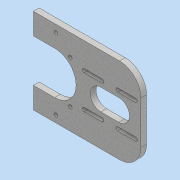
# Autodesk Inventor part: Uchwyt silnika krokowego osi Zi
Saved by Autodesk Inventor 2018 (Build 220112000, 112)
## iProperties
Created: 2019-02-03
Part Number: Uchwyt silnika krokowego osi Zi
Material: Ogólny
Document SubType Name: Modeling
Designer: Dawid
Density: 1 g/cm^3
Appearance: Aluminium odlewane
Author: Dawid
Autodesk Inventor part; units mm, degrees
ref_plane "YZ Plane" through (0, 0, 0) normal (1, 0, 0) x (0, 1, 0)
ref_plane "XZ Plane" through (0, 0, 0) normal (0, 1, 0) x (-1, 0, 0)
ref_plane "XY Plane" through (0, 0, 0) normal (0, 0, 1) x (1, 0, 0)
sketch "Szkic1" plane through (0, 0, 0) normal (0, 1, 0) x (-1, 0, 0)
  line L0 (-28, -60) -> (29, -60)
  line L1 (-28, 60) -> (29, 60)
  line L2 (-28, 60) -> (-36, 60)
  line L3 (-36, -60) -> (-28, -60)
  circle A0 centre (-81, 0) radius 12.5
  circle A1 centre (0, 0) radius 24
  line L4 (-111, -60) -> (-36, -60)
  line L5 (-111, 60) -> (-36, 60)
  line L6 (29, 60) -> (29, -60)
  line L7 (-31, -30) -> (29, -30)
  line L8 (-31, 30) -> (29, 30)
  circle A2 centre (-81, 0) radius 15
  line L9 (-116, -60) -> (-111, -60)
  line L10 (-116, 60) -> (-111, 60)
  line L11 (-116, -60) -> (-119.57, -60)
  line L12 (-119.57, 60) -> (-116, 60)
  line L13 (-119.57, -60) -> (-122.07, -60)
  line L14 (-122.07, -60) -> (-122.07, 60)
  line L15 (-122.07, 60) -> (-119.57, 60)
  line L16 (-31, -30) -> (-31, 30)
  dimension "d0" = 30
  constraints: 34 end point, 4 perpendicular, 3 centre point, 3 horizontal, 2 point on line, 1 coincident, 1 collinear, 1 vertical
  measures "d0" diameter of A2
extrude "Wyciągnięcie proste1" add sketch "Szkic1" along normal blind 8 contours L3 L4 L9 L11 L13 L14 L15 L12 L10 L5 L2 L1 L6 L8 L16 L7 L0
sketch "Szkic3" plane through (0, 8, 0) normal (0, 1, 0) x (1, 0, 0)
  line L0 (81, 15) -> (111, 15)
  line L1 (81, -15) -> (111, -15)
  arc A0 (11, -30) -> (11, 30) centre (11, 0) ccw projected
  circle A1 centre (81, 0) radius 15 projected
  arc A2 (66, 15) -> (66, -15) centre (66, 0) ccw
  line L2 (81, 15) -> (66, 15)
  line L3 (81, -15) -> (66, -15)
  arc A3 (91, -15) -> (91, 15) centre (91, 0) ccw
  line L4 (116, -60) -> (116, 60) projected
  line L5 (111, 15) -> (116, 15)
  line L6 (111, -15) -> (116, -15)
  point P0 (0, 0)
  point P1 (116, -30)
  point P2 (116, 30)
  constraints: 12 end point, 5 point on circle, 5 point on line, 2 centre point, 2 perpendicular, 1 parallel, 1 tangent
extrude "Wyciągnięcie proste4" cut sketch "Szkic3" against normal up to next contours L0 A3 L1 A1 | A1 | A1 L3 A2 L2
sketch "Szkic4" plane through (0, 8, 0) normal (0, 1, 0) x (1, 0, 0)
  line L0 (86, -60) -> (-29, -60)
  line L1 (-29, -60) -> (-29, -30)
  line L2 (-29, -30) -> (11, -30)
  arc A0 (11, -30) -> (11, 30) centre (11, 0) ccw
  line L3 (11, 30) -> (-29, 30)
  line L4 (-29, 30) -> (-29, 60)
  line L5 (-29, 60) -> (86, 60)
  circle A1 centre (81, 0) radius 4
  circle A2 centre (0, 0) radius 5
  circle A3 centre (104.57, -23.57) radius 2.5
  circle A4 centre (57.43, -23.57) radius 2.5
  circle A5 centre (104.57, 23.57) radius 2.5
  circle A6 centre (57.43, 23.57) radius 2.5
  line L6 (122.07, 60) -> (-29, 60) projected
  line L7 (-29, 60) -> (-29, 30) projected
  line L8 (104.57, 23.57) -> (114.57, 23.57)
  line L9 (104.57, 23.57) -> (89.57, 23.57)
  arc A7 (114.57, 21.07) -> (114.57, 26.07) centre (114.57, 23.57) ccw
  arc A8 (89.57, 26.07) -> (89.57, 21.07) centre (89.57, 23.57) ccw
  line L10 (104.57, 26.07) -> (114.57, 26.07)
  line L11 (104.57, 21.07) -> (114.57, 21.07)
  line L12 (104.57, 26.07) -> (89.57, 26.07)
  line L13 (104.57, 21.07) -> (89.57, 21.07)
  circle A9 centre (104.57, -23.57) radius 2.5
  line L14 (104.57, -23.57) -> (114.57, -23.57)
  line L15 (104.57, -23.57) -> (89.57, -23.57)
  arc A10 (114.57, -26.07) -> (114.57, -21.07) centre (114.57, -23.57) ccw
  arc A11 (89.57, -21.07) -> (89.57, -26.07) centre (89.57, -23.57) ccw
  line L16 (104.57, -21.07) -> (114.57, -21.07)
  line L17 (104.57, -26.07) -> (114.57, -26.07)
  line L18 (104.57, -21.07) -> (89.57, -21.07)
  line L19 (104.57, -26.07) -> (89.57, -26.07)
  circle A12 centre (57.43, -23.57) radius 2.5
  line L20 (57.43, -23.57) -> (67.43, -23.57)
  line L21 (57.43, -23.57) -> (42.43, -23.57)
  arc A13 (67.43, -26.07) -> (67.43, -21.07) centre (67.43, -23.57) ccw
  arc A14 (42.43, -21.07) -> (42.43, -26.07) centre (42.43, -23.57) ccw
  line L22 (57.43, -21.07) -> (67.43, -21.07)
  line L23 (57.43, -26.07) -> (67.43, -26.07)
  line L24 (57.43, -21.07) -> (42.43, -21.07)
  line L25 (57.43, -26.07) -> (42.43, -26.07)
  circle A15 centre (57.43, 23.57) radius 2.5
  line L26 (57.43, 23.57) -> (67.43, 23.57)
  line L27 (57.43, 23.57) -> (42.43, 23.57)
  arc A16 (67.43, 21.07) -> (67.43, 26.07) centre (67.43, 23.57) ccw
  arc A17 (42.43, 26.07) -> (42.43, 21.07) centre (42.43, 23.57) ccw
  line L28 (57.43, 26.07) -> (67.43, 26.07)
  line L29 (57.43, 21.07) -> (67.43, 21.07)
  line L30 (57.43, 26.07) -> (42.43, 26.07)
  line L31 (57.43, 21.07) -> (42.43, 21.07)
  point P0 (0, 0)
  point P1 (86, 60)
  point P2 (116, 60)
  point P3 (119.57, 60)
  dimension "d17" = 10
  dimension "d18" = 15
  dimension "d20" = 2.5
  dimension "d22" = 10
  dimension "d23" = 15
  dimension "d24" = 2.5
  dimension "d25" = 10
  dimension "d26" = 15
  dimension "d27" = 2.5
  dimension "d28" = 10
  dimension "d29" = 15
  dimension "d30" = 2.5
  constraints: 60 end point, 26 point on circle, 18 centre point, 12 horizontal, 12 parallel, 8 coincident, 8 tangent
  measures "d17" distance of L8.start L8.end
  measures "d18" distance of L8.start L9.end
  measures "d20" radius of A8
  measures "d22" distance of L15.start L14.end
  measures "d23" distance of L15.start L15.end
  measures "d24" radius of A11
  measures "d25" distance of L21.start L20.end
  measures "d26" distance of L21.start L21.end
  measures "d27" radius of A14
  measures "d28" distance of L27.start L26.end
  measures "d29" distance of L27.start L27.end
  measures "d30" radius of A17
extrude "Wyciągnięcie proste5" cut sketch "Szkic4" against normal up to next contours L14 L15 A3 | A3 L16 A10 L17 | A3 L15 L14 | A3 L19 A11 L18 | L20 L21 A4 | A4 L22 A13 L23 | A4 L21 L20 | A4 L25 A14 L24 | L8 L9 A5 | A5 L10 A7 L11 | A5 L9 L8 | A5 L13 A8 L12 | L26 L27 A6 | A6 L28 A16 L29 | A6 L27 L26 | A6 L31 A17 L30
fillet "Zaokrąglenie5" radius 30 2 edges at (31, 4, -30) (31, 4, 30)
fillet "Zaokrąglenie6" radius 30 2 edges at (122.07, 4, 60) (122.07, 4, -60)
sketch "Szkic5" plane through (0, 0, 0) normal (0, -1, 0) x (1, 0, 0)
  line L0 (122.07, 30) -> (122.07, -30)
  arc A0 (122.07, 30) -> (92.07, 60) centre (92.07, 30) ccw
  line L1 (-29, 60) -> (92.07, 60)
  line L2 (-29, 30) -> (-29, 60)
  arc A1 (1, -30) -> (1, 30) centre (1, 0) ccw
  line L3 (1, 30) -> (-29, 30)
  line L4 (-29, -30) -> (1, -30)
  line L5 (-29, -60) -> (-29, -30)
  line L6 (92.07, -60) -> (-29, -60)
  arc A2 (92.07, -60) -> (122.07, -30) centre (92.07, -30) ccw
  circle A3 centre (0, 0) radius 24
  arc A4 (-16.7697, 48.5) -> (-16.7697, 51.5) centre (-12, 50) ccw
  circle A5 centre (-19, 16) radius 2.5
  line L7 (-16.7697, 48.5) -> (-29, 48.5)
  line L8 (-29, 51.5) -> (-16.7697, 51.5)
  circle A6 centre (-12, -50) radius 5
  line L9 (-29, -48.5) -> (-16.7697, -48.5)
  line L10 (-16.7697, -51.5) -> (-29, -51.5)
  circle A7 centre (-19, -16) radius 2.5
  line L11 (36, -60) -> (36, 60)
  line L12 (-29, 60) -> (92.07, 60) projected
  line L13 (-29, 30) -> (-29, 60) projected
  line L14 (36, 60) -> (28, 60)
  line L15 (28, 60) -> (28, -60)
  line L16 (92.07, -60) -> (-29, -60) projected
  line L17 (28, -60) -> (18, -60)
  line L18 (18, -60) -> (18, 60)
  line L19 (18, -60) -> (18, -30)
  line L20 (18, 60) -> (18, 30)
  circle A8 centre (18, 30) radius 2.5
  circle A9 centre (18, -30) radius 2.5
  line L21 (18, -60) -> (3, -60)
  line L22 (3, -60) -> (3, 60)
  line L23 (3, 60) -> (3, 50)
  line L24 (3, -60) -> (3, -50)
  circle A10 centre (3, 50) radius 2.5
  circle A11 centre (3, -50) radius 2.5
  line L25 (28, -60) -> (23, -60)
  line L26 (92.07, -60) -> (-29, -60) projected
  line L27 (23, -60) -> (23, 60)
  line L28 (-29, 60) -> (92.07, 60) projected
  circle A12 centre (23, 30) radius 2.5
  circle A13 centre (23, -30) radius 2.5
  point P0 (0, 0)
  dimension "d36" = 8
  dimension "d37" = 10
  dimension "d38" = 30
  dimension "d39" = 30
  dimension "d40" = 5
  dimension "d41" = 5
  dimension "d42" = 15
  dimension "d43" = 10
  dimension "d44" = 10
  dimension "d45" = 5
  dimension "d46" = 5
  dimension "d49" = 5
  dimension "d50" = 5
  dimension "d51" = 5
  constraints: 48 end point, 14 centre point, 13 point on line, 8 point on circle, 4 coincident, 4 perpendicular, 2 other
  measures "d36" distance of L11.end L14.end
  measures "d37" distance of L15.end L17.end
  measures "d38" distance of L17.end L19.end
  measures "d39" distance of L18.end L20.end
  measures "d40" diameter of A8
  measures "d41" diameter of A9
  measures "d42" distance of L17.end L21.end
  measures "d43" distance of L22.end L23.end
  measures "d44" distance of L21.end L24.end
  measures "d45" diameter of A10
  measures "d46" diameter of A11
  measures "d49" distance of L15.end L25.end
  measures "d50" diameter of A12
  measures "d51" diameter of A13
extrude "Wyciągnięcie proste7" cut sketch "Szkic5" against normal up to next contours A12 L27 | L27 A12 | A13 L27 | L27 A13 | A10 L22 | L22 A10 | A11 L22 | L22 A11
